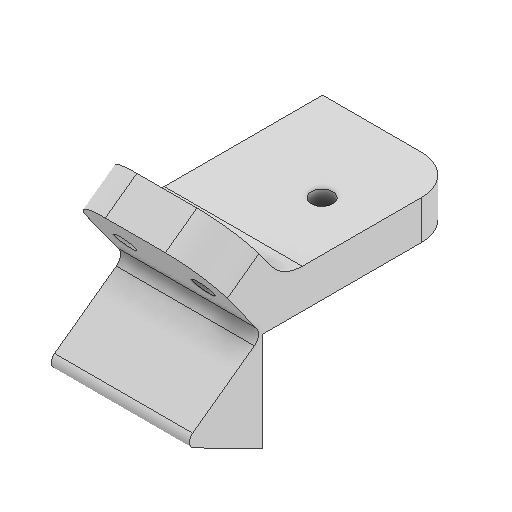
# Autodesk Inventor part: lowerRearBracket
Saved by Autodesk Inventor 2025 (Build 290162000, 162)
## iProperties
Created: 2024-12-14
Part Number: lowerRearBracket
Material: Generic
Document SubType Name: Modeling
Designer: derm
Density: 1 g/cm^3
Appearance: Default
Author: derm
Autodesk Inventor part; units mm, degrees
ref_plane "YZ Plane" through (0, 0, 0) normal (1, 0, 0) x (0, 1, 0)
ref_plane "XZ Plane" through (0, 0, 0) normal (0, 1, 0) x (-1, 0, 0)
ref_plane "XY Plane" through (0, 0, 0) normal (0, 0, 1) x (1, 0, 0)
sketch "Sketch1" plane through (0, 0, 0) normal (1, 0, 0) x (0, 1, 0)
  line L0 (0, 0) -> (25.4, 0)
  line L1 (25.4, 0) -> (25.4, -50.8)
  line L2 (25.4, -50.8) -> (0, -50.8)
  line L3 (0, -50.8) -> (0, 0)
  circle A0 centre (12.7, -12.9077) radius 2.75
  circle A1 centre (12.7, -40.4254) radius 2.75
  dimension "d0" = 25.4
  dimension "d1" = 50.8
  dimension "d2" = 5.5
  dimension "d3" = 5.5
  constraints: 8 end point, 2 centre point, 2 parallel, 1 horizontal, 1 perpendicular
  measures "d0" distance between parallel lines of L3 L1
  measures "d1" distance of L0.end L1.end
  measures "d2" diameter of A1
  measures "d3" diameter of A0
extrude "Extrusion1" add sketch "Sketch1" along normal blind 10
sketch "Sketch2" plane through (0, 0, 0) normal (-1, 0, 0) x (0, 0, 1)
  line L0 (-50.8, 0) -> (-50.8, 25.4)
  line L1 (0, 0) -> (-50.8, 0)
  line L2 (0, 25.4) -> (0, 0)
  line L3 (-50.8, 25.4) -> (0, 25.4)
  circle A0 centre (-40.4254, 12.7) radius 2.75
  circle A1 centre (-12.9077, 12.7) radius 2.75
  line L4 (2.3448, 23.6998) -> (5.142, 21.6715)
  line L5 (3.7285, 30.542) -> (1.7002, 27.7448)
  line L6 (20.0524, 42.2345) -> (17.2552, 44.2628)
  line L7 (22.2632, 12.8343) -> (24.2915, 15.6316)
  line L8 (15.4211, 14.2181) -> (18.2183, 12.1898)
  line L9 (0, 25.4) -> (14.9104, 45.963)
  line L10 (14.9104, 45.963) -> (6.8148, 51.8333)
  line L11 (-12.3523, 25.4) -> (6.8148, 51.8333)
  line L12 (0, 25.4) -> (20.563, 10.4896)
  line L13 (20.563, 10.4896) -> (0, 0)
  line L14 (-50.8, 25.4) -> (0, 25.4)
  line L15 (0, 25.4) -> (0, 35.4)
  line L16 (0, 35.4) -> (-50.8, 35.4)
  line L17 (-50.8, 35.4) -> (-50.8, 25.4)
  arc A2 (1.1565, 26.7905) -> (1.5314, 24.4378) centre (3.607, 25.9748) ccw
  arc A3 (1.5161, 27.4909) -> (2.0909, 23.8839) centre (3.607, 25.9748) ccw
  point P0 (-5.1012, 35.4)
  point P1 (1.5314, 24.4378)
  point P2 (1.1565, 26.7905)
extrude "Extrusion2" add sketch "Sketch2" against normal blind 35.4 contours L17 L16 L11 L3 | L2 L12 L4 L8 L13 | L11 L16 L15 L3 | L15 L16 L11 L10 L9 L5 | L9 A3 A2 L12
sketch "Sketch3" plane through (0, 35.4, -5.1012) normal (0, 1, 0) x (1, 0, 0)
  line L0 (0, 0) -> (0, 45.6988) projected
  line L1 (0, 0) -> (35.4, 0) projected
  line L2 (35.4, 45.6988) -> (35.4, 0) projected
  line L3 (0, 45.6988) -> (35.4, 45.6988) projected
  line L4 (10, 45.6988) -> (10, -5.1012) projected
  line L5 (10, 45.6988) -> (35.4, 45.6988) projected
  line L6 (35.4, -5.1012) -> (35.4, 45.6988) projected
  line L7 (10, -5.1012) -> (35.4, -5.1012) projected
  line L8 (10, 38.0742) -> (10, 32.5742) projected
  line L9 (10, 45.6988) -> (10, -5.1012) projected
  line L10 (10, -5.1012) -> (10, 45.6988) projected
  line L11 (10, 38.0742) -> (10, 32.5742) projected
  line L12 (10, 10.5565) -> (10, 5.0565) projected
  circle A0 centre (22.7, 22.8494) radius 2.75
  point P0 (0, -5.1012)
  dimension "d10" = 5.5
  constraints: 1 centre point
  measures "d10" diameter of A0
extrude "Extrusion3" cut sketch "Sketch3" against normal blind 35.4 contours A0
sketch "Sketch4" plane through (0, 27.4909, 1.5161) normal (0, -0.587, 0.8096) x (1, 0, 0)
  line L0 (0, -2.5827) -> (35.4, -2.5827) projected
  line L1 (0, 22.8173) -> (35.4, 22.8173) projected
  line L2 (0, 22.8173) -> (0, 2.5185) projected
  line L3 (0, 22.8173) -> (0, -2.5827) construction
  line L4 (7.7, 10.1173) -> (27.7, 10.1173) construction
  line L5 (7.7, 7.5173) -> (27.7, 7.5173)
  line L6 (27.7, 12.7173) -> (7.7, 12.7173)
  arc A0 (7.7, 12.7173) -> (7.7, 7.5173) centre (7.7, 10.1173) ccw
  arc A1 (27.7, 7.5173) -> (27.7, 12.7173) centre (27.7, 10.1173) ccw
  circle A2 centre (7.7, 10.1173) radius 2.6
  circle A3 centre (27.7, 10.1173) radius 2.6
  point P0 (0, -23.1457)
  point P1 (17.7, 10.1173)
  dimension "d13" = 2.6
  dimension "d14" = 20
  constraints: 10 end point, 4 point on circle, 4 tangent, 2 centre point, 2 coincident, 1 collinear, 1 horizontal, 1 midpoint, 1 parallel, 7 other
  measures "d13" radius of A1
  measures "d14" distance of L4.start L4.end
extrude "Extrusion4" cut sketch "Sketch4" against normal blind 35.4 contours A0 A2 | A3 A1
fillet "Fillet1" radius 10 1 edges at (17.7, 35.4, -5.1012)
fillet "Fillet2" radius 10 4 edges at (0, 48.8982, 10.8626) (35.4, 48.8982, 10.8626) (35.4, 30.4, -50.8) (5, 0, -50.8)
fillet "Fillet3" radius 2 1 edges at (17.7, 10.4896, 20.563)
body "Solid1"
